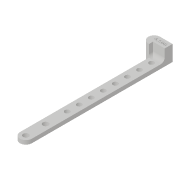
# Autodesk Inventor part: CollectorArmRear4_525long
Saved by Autodesk Inventor 2018 (Build 220112000, 112)
## iProperties
Created: 2019-02-19
Part Number: CollectorArmRear4_525long
Material: Generic
Document SubType Name: Modeling
Designer: ball
Density: 1 g/cm^3
Appearance: Default
Author: ball
Autodesk Inventor part; units mm, degrees
ref_plane "YZ Plane" through (0, 0, 0) normal (1, 0, 0) x (0, 1, 0)
ref_plane "XZ Plane" through (0, 0, 0) normal (0, 1, 0) x (-1, 0, 0)
ref_plane "XY Plane" through (0, 0, 0) normal (0, 0, 1) x (1, 0, 0)
sketch "Sketch1" plane through (0, 0, 0) normal (0, 1, 0) x (-1, 0, 0)
  line L0 (0, 0) -> (10.16, 0)
  line L1 (9.525, 9.6012) -> (9.525, 114.3)
  line L2 (0, 114.3) -> (0, 0)
  circle A0 centre (4.7625, 114.3) radius 2.2479
  circle A1 centre (4.7625, 98.298) radius 2.2479
  circle A2 centre (4.7625, 80.7466) radius 1.9685
  arc A3 (10.16, 0) -> (10.16, 9.6012) centre (10.16, 4.8006) ccw
  line L3 (10.16, 9.6012) -> (9.525, 9.6012)
  circle A4 centre (4.7625, 70.9676) radius 1.9685
  circle A5 centre (4.7625, 61.1886) radius 1.9685
  circle A6 centre (4.7625, 51.4096) radius 1.9685
  circle A7 centre (4.7625, 41.6306) radius 1.9685
  circle A8 centre (4.7625, 31.8516) radius 1.9685
  circle A9 centre (4.7625, 22.0726) radius 1.9685
  circle A10 centre (4.7625, 12.2936) radius 1.9685
  arc A11 (9.525, 114.3) -> (0, 114.3) centre (4.7625, 114.3505) ccw
  dimension "d0" = 9.525
  dimension "d4" = 4.4958
  dimension "d5" = 4.4958
  dimension "d6" = 16.002
  dimension "d7" = 3.937
  dimension "d8" = 17.5514
  dimension "d16" = 4.8006
  dimension "d17" = 10.16
  dimension "d18" = 114.3
  dimension "d21" = 9.779
  dimension "d27" = 4.7628
  dimension "d28" = 0
  dimension "d29" = 0
  constraints: 12 centre point, 8 end point, 4 point on circle, 2 perpendicular, 1 coincident, 1 horizontal, 1 parallel, 1 vertical, 14 other
  measures "d0" distance of L2.start L1.end
  measures "d4" diameter of A0
  measures "d5" diameter of A1
  measures "d6" distance of A1.centre A0.centre
  measures "d7" diameter of A2
  measures "d8" distance of A2.centre A1.centre
  measures "d16" distance from line of L0 point (10.16, 4.801)
  measures "d17" distance from line of L2 point (10.16, 4.801)
  measures "d18" distance from line of L0 A0.centre
  measures "d21" distance of A2.centre A4.centre
  measures "d27" radius of A11
  measures "d28" vertical distance of L1.end A0.centre
  measures "d29" vertical distance of L2.start A0.centre
extrude "Extrusion1" add sketch "Sketch1" along normal blind 3.175
sketch "Sketch2" plane through (0, 3.175, 0) normal (0, 1, 0) x (1, 0, 0)
  line L0 (-9.525, -9.6012) -> (-9.525, -6.35)
  line L1 (-9.525, -6.35) -> (0, -6.35)
  line L2 (0, -114.3) -> (0, 0) projected
  line L3 (0, -6.35) -> (0, 0)
  arc A0 (-10.16, 0) -> (-10.16, -9.6012) centre (-10.16, -4.8006) ccw projected
  arc A1 (-10.16, 0) -> (-10.239, -9.6012) centre (-10.1597, -4.8009) ccw
  line L4 (-10.16, -9.6012) -> (-9.525, -9.6012) projected
  line L5 (-9.525, -9.6012) -> (-10.16, -9.6012)
  line L6 (0, 0) -> (-10.16, 0) projected
  line L7 (-10.16, 0) -> (0, 0)
  constraints: 10 end point, 3 point on circle, 2 perpendicular, 1 centre point, 1 collinear, 1 horizontal, 1 vertical
extrude "Extrusion2" add sketch "Sketch2" along normal blind 9.525
fillet "Fillet1" radius 3.175 2 edges at (-4.7625, 3.175, 6.35) (-9.525, 3.175, 7.9756)
sketch "Sketch5" plane through (0, 12.7, 0) normal (0, 1, 0) x (1, 0, 0)
  line L0 (-11.1912, 0.0281) -> (-1.5184, 0.0281) construction
  line L1 (-1.5184, 0.0281) -> (-1.5184, -6.3829) construction
  line L2 (-1.5184, -6.3829) -> (-11.1912, -6.3829) construction
  line L3 (-11.1912, -6.3829) -> (-11.1912, 0.0281) construction
  line L4 (-9.1953, -3.8536) -> (-9.5391, -3.8536)
  line L5 (-9.5391, -3.8536) -> (-9.5391, -4.4525)
  line L6 (-9.5391, -4.4525) -> (-10.1545, -4.4525)
  line L7 (-10.1545, -4.4525) -> (-10.1545, -3.8536)
  line L8 (-10.1545, -3.8536) -> (-11.2742, -3.8536)
  line L9 (-11.2742, -3.8536) -> (-11.2742, -3.3801)
  line L10 (-11.2742, -3.3801) -> (-10.1751, -1.9064)
  line L11 (-10.1751, -1.9064) -> (-9.5391, -1.9064)
  line L12 (-9.5391, -1.9064) -> (-9.5391, -3.3966)
  line L13 (-9.5391, -3.3966) -> (-9.1953, -3.3966)
  line L14 (-9.1953, -3.3966) -> (-9.1953, -3.8536)
  line L15 (-10.1545, -3.3966) -> (-10.1545, -2.5321)
  line L16 (-10.1545, -2.5321) -> (-10.7988, -3.3966)
  line L17 (-10.7988, -3.3966) -> (-10.1545, -3.3966)
  line L18 (-8.2793, -4.4464) -> (-8.8824, -4.4464)
  line L19 (-8.8824, -4.4464) -> (-8.8824, -3.7753)
  line L20 (-8.8824, -3.7753) -> (-8.2793, -3.7753)
  line L21 (-8.2793, -3.7753) -> (-8.2793, -4.4464)
  spline S0 degree 2 poles (-5.9678, -3.586) (-5.9678, -3.7856) (-6.1037, -4.1232) (-6.2375, -4.2446) knots 0 0 0 1 2 2 2
  spline S1 degree 2 poles (-6.2375, -4.2446) (-6.3713, -4.3661) (-6.7376, -4.4999) (-7.0052, -4.4999) knots 0 0 0 1 2 2 2
  spline S2 degree 2 poles (-7.0052, -4.4999) (-7.2893, -4.4978) (-7.6968, -4.4052) (-7.8306, -4.3455) knots 0 0 0 1 2 2 2
  line L22 (-7.8306, -4.3455) -> (-7.8306, -3.7918)
  line L23 (-7.8306, -3.7918) -> (-7.773, -3.7918)
  spline S3 degree 2 poles (-7.773, -3.7918) (-7.7236, -3.8186) (-7.6042, -3.8886) (-7.5075, -3.9256) knots 0 0 0 1 2 2 2
  spline S4 degree 2 poles (-7.5075, -3.9256) (-7.4169, -3.9606) (-7.2296, -4.0079) (-7.1164, -4.0079) knots 0 0 0 1 2 2 2
  spline S5 degree 2 poles (-7.1164, -4.0079) (-7.0176, -4.0079) (-6.787, -3.9585) (-6.7171, -3.8927) knots 0 0 0 1 2 2 2
  spline S6 degree 2 poles (-6.7171, -3.8927) (-6.6656, -3.8412) (-6.608, -3.7157) (-6.608, -3.6107) knots 0 0 0 1 2 2 2
  spline S7 degree 2 poles (-6.608, -3.6107) (-6.608, -3.5201) (-6.6821, -3.3925) (-6.7418, -3.3534) knots 0 0 0 1 2 2 2
  spline S8 degree 2 poles (-6.7418, -3.3534) (-6.8282, -3.2958) (-7.0752, -3.2628) (-7.1637, -3.2628) knots 0 0 0 1 2 2 2
  spline S9 degree 2 poles (-7.1637, -3.2628) (-7.3037, -3.2628) (-7.5692, -3.3081) (-7.666, -3.3328) knots 0 0 0 1 2 2 2
  line L24 (-7.666, -3.3328) -> (-7.7215, -3.3328)
  line L25 (-7.7215, -3.3328) -> (-7.7215, -1.9064)
  line L26 (-7.7215, -1.9064) -> (-6.0378, -1.9064)
  line L27 (-6.0378, -1.9064) -> (-6.0378, -2.386)
  line L28 (-6.0378, -2.386) -> (-7.1184, -2.386)
  line L29 (-7.1184, -2.386) -> (-7.1184, -2.8079)
  spline S10 degree 2 poles (-7.1184, -2.8079) (-7.067, -2.8038) (-6.925, -2.7997) (-6.8858, -2.7997) knots 0 0 0 1 2 2 2
  spline S11 degree 2 poles (-6.8858, -2.7997) (-6.7027, -2.7997) (-6.3939, -2.8738) (-6.2725, -2.9499) knots 0 0 0 1 2 2 2
  spline S12 degree 2 poles (-6.2725, -2.9499) (-6.1284, -3.0446) (-5.9678, -3.3596) (-5.9678, -3.586) knots 0 0 0 1 2 2 2
  spline S13 degree 2 poles (-3.7181, -3.1764) (-3.7181, -3.5057) (-3.823, -3.9997) (-3.9404, -4.1664) knots 0 0 0 1 2 2 2
  spline S14 degree 2 poles (-3.9404, -4.1664) (-4.0556, -4.3311) (-4.4282, -4.4999) (-4.6958, -4.4999) knots 0 0 0 1 2 2 2
  spline S15 degree 2 poles (-4.6958, -4.4999) (-4.9654, -4.4999) (-5.3359, -4.3311) (-5.4532, -4.1623) knots 0 0 0 1 2 2 2
  spline S16 degree 2 poles (-5.4532, -4.1623) (-5.5706, -3.9956) (-5.6755, -3.5057) (-5.6755, -3.1764) knots 0 0 0 1 2 2 2
  spline S17 degree 2 poles (-5.6755, -3.1764) (-5.6755, -2.8388) (-5.5706, -2.3613) (-5.4512, -2.1884) knots 0 0 0 1 2 2 2
  spline S18 degree 2 poles (-5.4512, -2.1884) (-5.3318, -2.0196) (-4.9551, -1.8549) (-4.6958, -1.8549) knots 0 0 0 1 2 2 2
  spline S19 degree 2 poles (-4.6958, -1.8549) (-4.422, -1.8549) (-4.0556, -2.0278) (-3.9383, -2.1987) knots 0 0 0 1 2 2 2
  spline S20 degree 2 poles (-3.9383, -2.1987) (-3.823, -2.3654) (-3.7181, -2.8573) (-3.7181, -3.1764) knots 0 0 0 1 2 2 2
  spline S21 degree 2 poles (-4.3582, -3.1764) (-4.3582, -2.705) (-4.5126, -2.3242) (-4.6958, -2.3242) knots 0 0 0 1 2 2 2
  spline S22 degree 2 poles (-4.6958, -2.3242) (-4.879, -2.3242) (-5.0354, -2.705) (-5.0354, -3.1784) knots 0 0 0 1 2 2 2
  spline S23 degree 2 poles (-5.0354, -3.1784) (-5.0354, -3.6436) (-4.879, -4.0306) (-4.6958, -4.0306) knots 0 0 0 1 2 2 2
  spline S24 degree 2 poles (-4.6958, -4.0306) (-4.5146, -4.0306) (-4.3582, -3.6436) (-4.3582, -3.1764) knots 0 0 0 1 2 2 2
  spline S25 degree 2 poles (-1.493, -3.1764) (-1.493, -3.5057) (-1.598, -3.9997) (-1.7153, -4.1664) knots 0 0 0 1 2 2 2
  spline S26 degree 2 poles (-1.7153, -4.1664) (-1.8305, -4.3311) (-2.2031, -4.4999) (-2.4707, -4.4999) knots 0 0 0 1 2 2 2
  spline S27 degree 2 poles (-2.4707, -4.4999) (-2.7403, -4.4999) (-3.1108, -4.3311) (-3.2282, -4.1623) knots 0 0 0 1 2 2 2
  spline S28 degree 2 poles (-3.2282, -4.1623) (-3.3455, -3.9956) (-3.4505, -3.5057) (-3.4505, -3.1764) knots 0 0 0 1 2 2 2
  spline S29 degree 2 poles (-3.4505, -3.1764) (-3.4505, -2.8388) (-3.3455, -2.3613) (-3.2261, -2.1884) knots 0 0 0 1 2 2 2
  spline S30 degree 2 poles (-3.2261, -2.1884) (-3.1067, -2.0196) (-2.73, -1.8549) (-2.4707, -1.8549) knots 0 0 0 1 2 2 2
  spline S31 degree 2 poles (-2.4707, -1.8549) (-2.1969, -1.8549) (-1.8305, -2.0278) (-1.7132, -2.1987) knots 0 0 0 1 2 2 2
  spline S32 degree 2 poles (-1.7132, -2.1987) (-1.598, -2.3654) (-1.493, -2.8573) (-1.493, -3.1764) knots 0 0 0 1 2 2 2
  spline S33 degree 2 poles (-2.1331, -3.1764) (-2.1331, -2.705) (-2.2875, -2.3242) (-2.4707, -2.3242) knots 0 0 0 1 2 2 2
  spline S34 degree 2 poles (-2.4707, -2.3242) (-2.6539, -2.3242) (-2.8103, -2.705) (-2.8103, -3.1784) knots 0 0 0 1 2 2 2
  spline S35 degree 2 poles (-2.8103, -3.1784) (-2.8103, -3.6436) (-2.6539, -4.0306) (-2.4707, -4.0306) knots 0 0 0 1 2 2 2
  spline S36 degree 2 poles (-2.4707, -4.0306) (-2.2896, -4.0306) (-2.1331, -3.6436) (-2.1331, -3.1764) knots 0 0 0 1 2 2 2
  point P0 (0, 0)
  constraints: 2 other
emboss "Emboss1" sketch "Sketch5" operation cut depth 0.762 direction (0, -1, 0)
body "Solid1"
